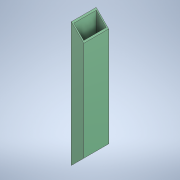
# Autodesk Inventor part: PerfilD2
Saved by Autodesk Inventor 2021 (Build 250183000, 183)
## iProperties
Created: 2021-06-11
Part Number: PerfilD2
Material: Generic
Document SubType Name: Modeling
Designer: lcper
Density: 1 g/cm^3
Appearance: Default
Author: lcper
Autodesk Inventor part; units mm, degrees
ref_plane "YZ Plane" through (0, 0, 0) normal (1, 0, 0) x (0, 1, 0)
ref_plane "XZ Plane" through (0, 0, 0) normal (0, 1, 0) x (-1, 0, 0)
ref_plane "XY Plane" through (0, 0, 0) normal (0, 0, 1) x (1, 0, 0)
sketch "Sketch1" plane through (0, 0, 0) normal (0, 1, 0) x (-1, 0, 0)
  line L0 (-9.4777, 15.0257) -> (40.5223, 15.0257)
  line L1 (40.5223, 15.0257) -> (40.5223, -84.9743)
  line L2 (40.5223, -84.9743) -> (-9.4777, -84.9743)
  line L3 (-9.4777, -84.9743) -> (-9.4777, 15.0257)
  line L4 (35.5223, 10.0257) -> (-4.4777, 10.0257)
  line L5 (-4.4777, 10.0257) -> (-4.4777, -79.9743)
  line L6 (-4.4777, -79.9743) -> (35.5223, -79.9743)
  line L7 (35.5223, -79.9743) -> (35.5223, 10.0257)
  point P0 (0, 0)
  point P1 (0, 0)
  dimension "d0" = 50
  dimension "d1" = 100
  dimension "d2" = 5
  dimension "d3" = 90
  dimension "d4" = 5
  dimension "d5" = 40
  constraints: 16 end point, 4 parallel, 2 horizontal, 2 perpendicular
  measures "d0" distance of L1.end L2.end
  measures "d1" distance of L0.end L1.end
  measures "d2" distance between parallel lines of L4 L0
  measures "d3" distance of L6.end L4.start
  measures "d4" distance between parallel lines of L1 L7
  measures "d5" distance of L5.end L6.end
extrude "Extrusion1" add sketch "Sketch1" along normal blind 500
sketch "Sketch2" plane through (-40.5223, 0, 15.0257) normal (0, 0, 1) x (1, 0, 0)
  line L0 (0, 0) -> (50, 0) projected
  line L1 (0, 0) -> (70.7251, 0) construction
  line L2 (45, 0) -> (45, 500) projected
  line L3 (0, 0) -> (50, 50)
  line L4 (50, 0) -> (50, 500) projected
  line L5 (0, 0) -> (70.7107, 0) construction
  line L6 (50, 50) -> (50, 0)
  line L7 (50, 0) -> (0, 0)
  line L8 (0, 0) -> (0, 500) projected
  line L9 (0, 500) -> (50, 450)
  line L10 (0, 500) -> (70.7107, 500) construction
  line L11 (50, 450) -> (50, 500)
  line L12 (50, 500) -> (0, 500)
  point P0 (40.5223, 0)
  dimension "d9" = 45
  dimension "d10" = 45
  constraints: 18 end point, 3 horizontal, 3 point on line, 2 collinear, 2 equal length, 1 perpendicular
  measures "d9" angle of L5 L3
  measures "d10" angle of L9 L10
extrude "Extrusion2" cut sketch "Sketch2" against normal blind 500 contours L3 L2 L0 | L2 L3 L4 L0 | L12 L2 L9 | L2 L12 L4 L9
body "Solid1"
